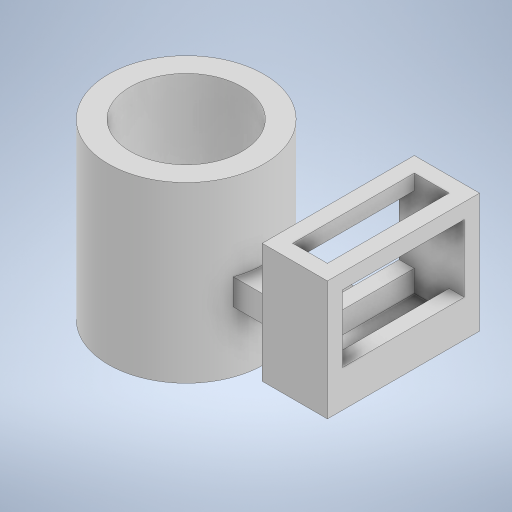
# Autodesk Inventor part: 카메라 거치대
Saved by Autodesk Inventor 2023 (Build 270158000, 158)
## iProperties
Created: 2022-10-20
Part Number: 카메라 거치대
Material: 일반
Document SubType Name: Sheet Metal
Designer: ghkdr
Density: 1 g/cm^3
Sheet Metal Rule: 기본값_mm
Appearance: 기본값
Author: ghkdr
Autodesk Inventor part; units mm, degrees
ref_plane "YZ Plane" through (0, 0, 0) normal (1, 0, 0) x (0, 1, 0)
ref_plane "XZ Plane" through (0, 0, 0) normal (0, 1, 0) x (-1, 0, 0)
ref_plane "XY Plane" through (0, 0, 0) normal (0, 0, 1) x (1, 0, 0)
sketch "스케치1" plane through (0, 0, 0) normal (0, 1, 0) x (-1, 0, 0)
  line L0 (-8, 28) -> (8, 28)
  line L1 (8, 28) -> (8, -28)
  line L2 (8, -28) -> (-8, -28)
  line L3 (-8, -28) -> (-8, 28)
  line L4 (-8, 28) -> (8, -28) construction
  line L5 (8, 28) -> (-8, -28) construction
  line L6 (15, -35) -> (15, 35)
  line L7 (15, 35) -> (-15, 35)
  line L8 (-15, 35) -> (-15, -35)
  line L9 (-15, -35) -> (15, -35)
  point P0 (0, 0)
  dimension "d0" = 16
  dimension "d1" = 56
  dimension "d2" = 7
  constraints: 20 end point, 4 parallel, 2 midpoint, 2 perpendicular, 1 horizontal, 3 other
  measures "d0" distance of L1.end L2.end
  measures "d1" distance of L0.end L1.end
  measures "d2" distance between parallel lines of L1 L6
extrude "돌출1" add sketch "스케치1" along normal blind 55 contours L0 L1 L2 L3 | L9 L8 L7 L6
sketch "스케치2" plane through (0, 55, 0) normal (0, 1, 0) x (1, 0, 0)
  line L0 (-15, 35) -> (-15, -35) projected
  line L1 (-15, -35) -> (15, -35) projected
  line L2 (-15, -35) -> (15, -35) projected
  line L3 (15, -35) -> (15, 35) projected
  line L4 (15, 35) -> (-15, 35) projected
  line L5 (-15, 35) -> (-15, -35) projected
  line L6 (8, 28) -> (8, -28)
  line L7 (8, -28) -> (-8, -28)
  line L8 (-8, -28) -> (-8, 28)
  line L9 (-8, 28) -> (8, 28)
  point P0 (0, 0)
  dimension "d5" = 7
  constraints: 8 end point, 3 other
  measures "d5" distance between parallel lines of L3 L6
extrude "돌출2" cut sketch "스케치2" against normal blind 48 contours L6 L7 L8 L9
sketch "스케치3" plane through (15, 0, 35) normal (1, 0, 0) x (0, 0, -1)
  line L0 (0, 0) -> (70, 0) projected
  line L1 (70, 0) -> (70, 55) projected
  line L2 (0, 55) -> (70, 55) projected
  line L3 (0, 0) -> (0, 55) projected
  line L4 (63, 48) -> (63, 17)
  line L5 (7, 17) -> (7, 48)
  line L6 (7, 48) -> (63, 48)
  line L7 (7, 17) -> (63, 17)
  point P0 (35, 0)
  point P1 (0, 27.5)
  dimension "d8" = 7
  dimension "d10" = 17
  dimension "d11" = 7
  dimension "d12" = 7
  dimension "d13" = 31
  constraints: 8 end point, 1 midpoint
  measures "d8" distance between parallel lines of L2 L6
  measures "d10" distance between parallel lines of L0 L7
  measures "d11" distance between parallel lines of L1 L4
  measures "d12" distance from line of point (0, 27.5) L5
  measures "d13" distance of L5.start L5.end
extrude "돌출3" cut sketch "스케치3" against normal blind 40 contours L4 L7 L5 L6
sketch "스케치4" plane through (0, 7, 0) normal (0, 1, 0) x (1, 0, 0)
  line L0 (8, -28) -> (-8, -28) projected
  line L1 (-8, -28) -> (-8, 28) projected
  line L2 (8, 28) -> (8, -28) projected
  line L3 (8, -28) -> (-8, -28) projected
  line L4 (8, -21) -> (-8, -21)
  point P0 (0, 0)
  dimension "d16" = 7
  constraints: 2 end point, 1 parallel
  measures "d16" distance between parallel lines of L0 L4
extrude "돌출4" cut sketch "스케치4" against normal blind 10
sketch "스케치6" plane through (-15, 0, -35) normal (-1, 0, 0) x (0, 0, 1)
  line L0 (0, 0) -> (70, 0) projected
  line L1 (35, 0) -> (35, 55)
  line L2 (7, 55) -> (63, 55) projected
  line L3 (23, 12) -> (47, 12)
  line L4 (47, 0) -> (47, 12)
  line L5 (23, 0) -> (23, 12)
  dimension "d20" = 12
  dimension "d21" = 12
  dimension "d22" = 12
  constraints: 8 end point, 3 parallel, 1 midpoint
  measures "d20" distance between parallel lines of L0 L3
  measures "d21" distance between parallel lines of L1 L4
  measures "d22" distance between parallel lines of L1 L5
extrude "돌출5" add sketch "스케치6" along normal blind 70
sketch "스케치7" plane through (-15, 12, 12) normal (0, 1, 0) x (1, 0, 0)
  line L0 (-70, 24) -> (-70, 0) projected
  circle A0 centre (-70, 12) radius 35.75
  point P0 (15, 12)
  dimension "d25" = 71.5
  constraints: 1 centre point, 1 midpoint
  measures "d25" diameter of A0
extrude "돌출6" add sketch "스케치7" along normal mid plane 80
sketch "스케치8" plane through (-85, 52, 0) normal (0, 1, 0) x (1, 0, 0)
  circle A0 centre (0, 0) radius 35.75 projected
  circle A1 centre (0, 0) radius 25.75
  point P0 (85, 0)
  dimension "d28" = 10
  constraints: 1 centre point
  measures "d28" radial gap between concentric circles of A0 A1
extrude "돌출7" cut sketch "스케치8" against normal blind 80 contours A1
equation "\"TransitionRadius\" = BendRadius"
equation "\"BendRadius\" = 0.5"
